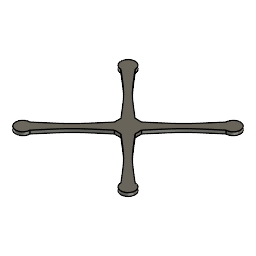
Drone 5 Polegadas (Autodesk Fusion 360 design; units mm, degrees)
Autodesk Fusion 360 part; units mm, degrees
sketch "Esboço1" plane through (0, 0, 0) normal (0, 0, 1) x (1, 0, 0)
  circle A0 centre (-78.5, 78.5) radius 10.65
  circle A1 centre (78.5, 78.5) radius 10.65
  circle A2 centre (-78.5, -78.5) radius 10.65
  circle A3 centre (78.5, -78.5) radius 10.65
  line L0 (-70.9693, 70.9693) -> (-15.4614, 15.4614)
  line L1 (-78.5, 0) -> (78.5, 0) construction
  line L2 (0, 78.5) -> (0, -78.5) construction
  line L3 (-70.9693, -70.9693) -> (-15.4614, -15.4614)
  line L4 (70.9693, 70.9693) -> (15.4614, 15.4614)
  line L5 (70.9693, -70.9693) -> (15.4614, -15.4614)
  line L6 (9.4614, -15.4614) -> (-9.4614, -15.4614)
  line L7 (-15.4614, -9.4614) -> (-15.4614, 9.4614)
  line L8 (-9.4614, 15.4614) -> (9.4614, 15.4614)
  line L9 (15.4614, 9.4614) -> (15.4614, -9.4614)
  line L10 (-46.9807, 36.3307) -> (-41.6557, 41.6557) construction
  line L11 (-36.3307, 46.9807) -> (-41.6557, 41.6557) construction
  spline S0 degree 2 poles (-78.5, 67.85) (-44.3182, 38.9932) (-15.4614, 4.8114) knots 0 0 0 8.932873 8.932873 8.932873 weights 1 3 1
  spline S1 degree 2 poles (-67.85, 78.5) (-38.9932, 44.3182) (-4.8114, 15.4614) knots 0 0 0 8.932873 8.932873 8.932873 weights 1 3 1
  spline S2 degree 2 poles (78.5, 67.85) (44.3182, 38.9932) (15.4614, 4.8114) knots 0 0 0 8.932873 8.932873 8.932873 weights 1 3 1
  spline S3 degree 2 poles (67.85, 78.5) (38.9932, 44.3182) (4.8114, 15.4614) knots 0 0 0 8.932873 8.932873 8.932873 weights 1 3 1
  spline S4 degree 2 poles (-78.5, -67.85) (-44.3182, -38.9932) (-15.4614, -4.8114) knots 0 0 0 8.932873 8.932873 8.932873 weights 1 3 1
  spline S5 degree 2 poles (-67.85, -78.5) (-38.9932, -44.3182) (-4.8114, -15.4614) knots 0 0 0 8.932873 8.932873 8.932873 weights 1 3 1
  spline S6 degree 2 poles (67.85, -78.5) (38.9932, -44.3182) (4.8114, -15.4614) knots 0 0 0 8.932873 8.932873 8.932873 weights 1 3 1
  spline S7 degree 2 poles (78.5, -67.85) (44.3182, -38.9932) (15.4614, -4.8114) knots 0 0 0 8.932873 8.932873 8.932873 weights 1 3 1
  arc A4 (-9.4614, 15.4614) -> (-15.4614, 9.4614) centre (-9.4614, 9.4614) ccw
  arc A5 (15.4614, 9.4614) -> (9.4614, 15.4614) centre (9.4614, 9.4614) ccw
  arc A6 (-15.4614, -9.4614) -> (-9.4614, -15.4614) centre (-9.4614, -9.4614) ccw
  arc A7 (9.4614, -15.4614) -> (15.4614, -9.4614) centre (9.4614, -9.4614) ccw
  dimension "d1" = 157
  dimension "d2" = 157
  dimension "d3" = 21.3
  dimension "d4" = 21.3
  dimension "d5" = 21.3
  dimension "d6" = 21.3
  dimension "d7" = 78.5
  dimension "d16" = 6
  dimension "d17" = 6
  constraint coincident A0 L0.start
  constraint symmetric L0.start L1 L3.start
  constraint symmetric L0.end L1 L3.end
  constraint symmetric L0.start L2 L4.start
  constraint symmetric L0.end L2 L4.end
  constraint symmetric L2 L3.start L5.start
  constraint symmetric L2 L3.end L5.end
  constraint horizontal L6
  constraint perpendicular L6 L7
  constraint parallel L6 L8
  constraint parallel L7 L9
  constraint coincident A0 S0.start
  constraint coincident L7 S0.end
  constraint coincident A0 S1.start
  constraint coincident L8 S1.end
  constraint coincident L0 L10.end
  constraint perpendicular L0 L10
  constraint perpendicular L0 L11
  constraint symmetric L2 S0.start S2.start
  constraint symmetric L2 S0.end S2.end
  constraint symmetric L2 S1.start S3.start
  constraint symmetric L2 S1.end S3.end
  constraint symmetric L2 S0 S2
  constraint symmetric L2 S1 S3
  constraint symmetric L1 S0.start S4.start
  constraint symmetric L1 S0.end S4.end
  constraint symmetric L1 S1.start S5.start
  constraint symmetric L1 S1.end S5.end
  constraint symmetric L1 S0 S4
  constraint symmetric L1 S1 S5
  constraint symmetric L1 S2.start S7.start
  constraint symmetric L1 S2.end S7.end
  constraint symmetric L1 S2 S7
  constraint symmetric L1 S3.start S6.start
  constraint symmetric L1 S3.end S6.end
  constraint symmetric L1 S3 S6
  constraint tangent L7 A4
  constraint tangent L8 A4
  constraint tangent L8 A5
  constraint tangent L9 A5
  constraint tangent L6 A6
  constraint tangent L7 A6
  constraint equal A5 A6
  constraint coincident L5.end L6
  constraint coincident L5.end L9
  constraint tangent L6 A7
  constraint tangent L9 A7
  constraint equal A5 A7
  measures "d1" distance of A0.centre A1.centre
  measures "d2" distance of A0.centre A2.centre
  measures "d3" diameter of A0
  measures "d4" diameter of A1
  measures "d5" diameter of A2
  measures "d6" diameter of A3
  measures "d7" distance of L0.start L0.end
  measures "d16" radius of A4
  measures "d17" radius of A5
extrude "Extrusão1" add sketch "Esboço1" along normal blind 5
equation "d8 = 0.75"
equation "d9 = 0.75"
equation "d10 = d8"
equation "d11 = d9"
equation "d12 = d8"
equation "d13 = d9"
equation "d14 = d11"
equation "d15 = d10"
